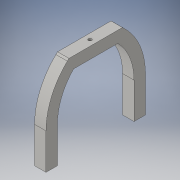
# Autodesk Inventor part: hpart
Saved by Autodesk Inventor 2016 (Build 200138000, 138)
## iProperties
Created: 2017-12-18
Part Number: hpart
Material: Generic
Document SubType Name: Modeling
Designer: student
Density: 1 g/cm^3
Appearance: Default
Author: student
Autodesk Inventor part; units mm, degrees
ref_plane "YZ Plane" through (0, 0, 0) normal (1, 0, 0) x (0, 1, 0)
ref_plane "XZ Plane" through (0, 0, 0) normal (0, 1, 0) x (-1, 0, 0)
ref_plane "XY Plane" through (0, 0, 0) normal (0, 0, 1) x (1, 0, 0)
sketch "Sketch1" plane through (0, 0, 0) normal (0, 1, 0) x (-1, 0, 0)
  line L0 (0, 34.29) -> (0, -34.29) construction
  line L1 (-4.445, 38.735) -> (4.445, 38.735)
  line L2 (4.445, 38.735) -> (4.445, 29.845)
  line L3 (4.445, 29.845) -> (-4.445, 29.845)
  line L4 (-4.445, 29.845) -> (-4.445, 38.735)
  line L5 (-4.445, 38.735) -> (4.445, 29.845) construction
  line L6 (4.445, 38.735) -> (-4.445, 29.845) construction
  line L7 (-4.445, -29.845) -> (4.445, -29.845)
  line L8 (4.445, -29.845) -> (4.445, -38.735)
  line L9 (4.445, -38.735) -> (-4.445, -38.735)
  line L10 (-4.445, -38.735) -> (-4.445, -29.845)
  line L11 (-4.445, -29.845) -> (4.445, -38.735) construction
  line L12 (4.445, -29.845) -> (-4.445, -38.735) construction
  point P0 (0, 0)
  point P1 (0, 0)
  dimension "d0" = 68.58
  dimension "d1" = 8.89
  dimension "d2" = 8.89
  dimension "d3" = 8.89
  constraints: 26 end point, 5 midpoint, 4 parallel, 2 coincident, 2 horizontal, 2 perpendicular, 1 point on line, 1 vertical
  measures "d0" distance of L0.start L0.end
  measures "d1" distance of L1.end L2.end
  measures "d2" distance of L1.start L1.end
  measures "d3" distance of L7.end L8.end
sketch "Sketch2" plane through (0, 0, 0) normal (1, 0, 0) x (0, 1, 0)
  line L0 (0, 0) -> (63.5, 0) construction
  line L1 (0, 34.29) -> (27.94, 34.29)
  line L2 (0, -34.29) -> (27.94, -34.29)
  line L3 (63.5, 19.05) -> (63.5, -19.05)
  arc A0 (63.5, 19.05) -> (27.94, 34.29) centre (27.94, -14.8167) ccw
  arc A1 (27.94, -34.29) -> (63.5, -19.05) centre (27.94, 14.8167) ccw
  dimension "d4" = 63.5
  dimension "d21" = 38.1
  dimension "d22" = 27.94
  dimension "d23" = 27.94
  constraints: 8 end point, 4 point on circle, 3 horizontal, 2 centre point, 2 tangent, 1 coincident, 1 horizontal alignment, 1 midpoint, 1 vertical
  measures "d4" distance of L0.start L0.end
  measures "d21" distance of L3.start L3.end
  measures "d22" distance of L1.start L1.end
  measures "d23" distance of L2.start L2.end
sweep "Sweep1" add profiles "Sketch1" path "Sketch2" contours L7 L8 L9 L10
sketch "Sketch3" plane through (-4.445, 0, -29.845) normal (0, -1, 0) x (1, 0, 0)
  line L0 (0, 0) -> (0, -8.89) projected
  circle A0 centre (4.445, -4.445) radius 1.27
  line L1 (0, 68.58) -> (0, 59.69) projected
  circle A1 centre (4.445, 64.135) radius 1.27
  point P0 (4.445, 29.845)
  dimension "d10" = 2.54
  dimension "d11" = 2.54
  dimension "d12" = 4.445
  dimension "d13" = 34.29
  dimension "d14" = 4.445
  dimension "d15" = 34.29
  constraints: 2 centre point
  measures "d10" diameter of A0
  measures "d11" diameter of A1
  measures "d12" distance from line of L0 A0.centre
  measures "d13" distance of point (4.445, 29.845) A0.centre
  measures "d14" distance from line of L1 A1.centre
  measures "d15" distance of point (4.445, 29.845) A1.centre
extrude "Extrusion1" cut sketch "Sketch3" against normal blind 8.89
sketch "Sketch5" plane through (-4.445, 67.945, 20.828) normal (0, 1, 0) x (1, 0, 0)
  circle A0 centre (4.445, 20.828) radius 1.27
  dimension "d24" = 2.54
  constraints: 1 centre point, 1 coincident
  measures "d24" diameter of A0
hole "Hole1" at (0, 67.945, 0) direction (0, -1, 0) diameter 2.54 end through all
body "Solid1"
